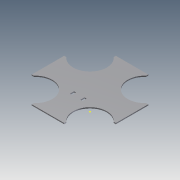
# Autodesk Inventor part: base bottom
Saved by Autodesk Inventor 2011 (Build 150239000, 239)
## iProperties
Created: 2011-07-30
Part Number: base bottom
Document SubType Name: Modeling
Designer: adowning
Density: 1 g/cm^3
Author: adowning
Autodesk Inventor part; units mm, degrees
ref_plane "YZ Plane" through (0, 0, 0) normal (1, 0, 0) x (0, 1, 0)
ref_plane "XZ Plane" through (0, 0, 0) normal (0, 1, 0) x (-1, 0, 0)
ref_plane "XY Plane" through (0, 0, 0) normal (0, 0, 1) x (1, 0, 0)
sketch "Sketch1" plane through (0, 0, 0) normal (0, 0, 1) x (1, 0, 0)
  point P0 (0, 0)
sketch "Sketch2" plane through (0, 0, 0) normal (0, 1, 0) x (-1, 0, 0)
  line L0 (-144.440152, 144.440152) -> (363.559848, 144.440152)
  line L1 (363.559848, 144.440152) -> (363.559848, -363.559848)
  line L2 (363.559848, -363.559848) -> (-144.440152, -363.559848)
  line L3 (-144.440152, -363.559848) -> (-144.440152, 144.440152)
  line L4 (363.559848, -363.559848) -> (274.659848, -363.559848)
  line L5 (274.659848, -363.559848) -> (274.659848, -274.659848)
  line L6 (274.659848, -274.659848) -> (363.559848, -274.659848)
  line L7 (363.559848, -274.659848) -> (363.559848, -363.559848)
  line L8 (-144.440152, -363.559848) -> (-55.540152, -363.559848)
  line L9 (-55.540152, -363.559848) -> (-55.540152, -274.659848)
  line L10 (-55.540152, -274.659848) -> (-144.440152, -274.659848)
  line L11 (-144.440152, -274.659848) -> (-144.440152, -363.559848)
  line L12 (-144.440152, 144.440152) -> (-55.540152, 144.440152)
  line L13 (-55.540152, 144.440152) -> (-55.540152, 55.540152)
  line L14 (-55.540152, 55.540152) -> (-144.440152, 55.540152)
  line L15 (-144.440152, 55.540152) -> (-144.440152, 144.440152)
  line L16 (363.559848, 144.440152) -> (274.659848, 144.440152)
  line L17 (274.659848, 144.440152) -> (274.659848, 55.540152)
  line L18 (274.659848, 55.540152) -> (363.559848, 55.540152)
  line L19 (363.559848, 55.540152) -> (363.559848, 144.440152)
  line L20 (363.559848, -363.559848) -> (173.059848, -363.559848)
  line L21 (173.059848, -363.559848) -> (173.059848, -173.059848)
  line L22 (173.059848, -173.059848) -> (363.559848, -173.059848)
  line L23 (363.559848, -173.059848) -> (363.559848, -363.559848)
  line L24 (-144.440152, -363.559848) -> (46.059848, -363.559848)
  line L25 (46.059848, -363.559848) -> (46.059848, -173.059848)
  line L26 (46.059848, -173.059848) -> (-144.440152, -173.059848)
  line L27 (-144.440152, -173.059848) -> (-144.440152, -363.559848)
  line L28 (-144.440152, 144.440152) -> (46.059848, 144.440152)
  line L29 (46.059848, 144.440152) -> (46.059848, -46.059848)
  line L30 (46.059848, -46.059848) -> (-144.440152, -46.059848)
  line L31 (-144.440152, -46.059848) -> (-144.440152, 144.440152)
  line L32 (363.559848, 144.440152) -> (173.059848, 144.440152)
  line L33 (173.059848, 144.440152) -> (173.059848, -46.059848)
  line L34 (173.059848, -46.059848) -> (363.559848, -46.059848)
  line L35 (363.559848, -46.059848) -> (363.559848, 144.440152)
  circle A0 centre (-55.540152, -274.659848) radius 101.6
  circle A1 centre (-55.540152, 55.540152) radius 101.6
  circle A2 centre (274.659848, 55.540152) radius 101.6
  circle A3 centre (274.659848, -274.659848) radius 101.6
  point P0 (0, 0)
  dimension "d0" = 508
  dimension "d1" = 508
  dimension "d2" = 88.9
  dimension "d3" = 88.9
  dimension "d4" = 88.9
  dimension "d5" = 88.9
  dimension "d6" = 88.9
  dimension "d7" = 88.9
  dimension "d8" = 88.9
  dimension "d9" = 88.9
  dimension "d10" = 190.5
  dimension "d11" = 190.5
  dimension "d12" = 190.5
  dimension "d13" = 190.5
  dimension "d14" = 190.5
  dimension "d15" = 190.5
  constraints: 72 end point, 18 parallel, 9 horizontal, 9 perpendicular, 4 centre point, 4 coincident, 4 tangent
  measures "d0" distance of L1.end L2.end
  measures "d1" distance of L0.end L1.end
  measures "d2" distance of L5.end L6.end
  measures "d3" distance of L4.end L5.end
  measures "d4" distance of L10.end L9.end
  measures "d5" distance of L9.end L8.end
  measures "d6" distance of L13.end L14.end
  measures "d7" distance of L12.end L13.end
  measures "d8" distance of L18.end L17.end
  measures "d9" distance of L17.end L16.end
  measures "d10" distance of L21.end L22.end
  measures "d11" distance of L20.end L21.end
  measures "d12" distance of L26.end L25.end
  measures "d13" distance of L25.end L24.end
  measures "d14" distance of L29.end L30.end
  measures "d15" distance of L28.end L29.end
extrude "Extrusion1" add sketch "Sketch2" along normal blind 12.7 contours L0 L33 L34 L1 L22 L21 L2 L25 L26 L3 L30 L29
fillet "Fillet1" radius 101.6 4 edges at (-173.0598, 6.35, -46.0598) (-46.0598, 6.35, -46.0598) (-46.0598, 6.35, -173.0598) (-173.0598, 6.35, -173.0598)
sketch "Sketch3" plane through (0, 12.7, 0) normal (0, 1, 0) x (1, 0, 0)
  line L0 (55.540152, 46.059848) -> (144.440152, 46.059848)
  line L1 (144.440152, 173.059848) -> (144.440152, 46.059848)
  line L2 (144.440152, 173.059848) -> (55.540152, 173.059848)
  arc A0 (-46.059848, 274.659848) -> (55.540152, 173.059848) centre (55.540152, 274.659848) ccw
  line L3 (-46.059848, 274.659848) -> (-46.059848, 363.559848)
  line L4 (-173.059848, 363.559848) -> (-46.059848, 363.559848)
  line L5 (-173.059848, 363.559848) -> (-173.059848, 274.659848)
  arc A1 (-274.659848, 173.059848) -> (-173.059848, 274.659848) centre (-274.659848, 274.659848) ccw
  line L6 (-274.659848, 173.059848) -> (-363.559848, 173.059848)
  line L7 (-363.559848, 46.059848) -> (-363.559848, 173.059848)
  line L8 (-363.559848, 46.059848) -> (-274.659848, 46.059848)
  arc A2 (-173.059848, -55.540152) -> (-274.659848, 46.059848) centre (-274.659848, -55.540152) ccw
  line L9 (-173.059848, -55.540152) -> (-173.059848, -144.440152)
  line L10 (-46.059848, -144.440152) -> (-173.059848, -144.440152)
  line L11 (-46.059848, -144.440152) -> (-46.059848, -55.540152)
  arc A3 (55.540152, 46.059848) -> (-46.059848, -55.540152) centre (55.540152, -55.540152) ccw
  circle A4 centre (55.540152, 274.659848) radius 101.6
  circle A5 centre (55.540152, -55.540152) radius 101.6
  circle A6 centre (-274.659848, -55.540152) radius 101.6
  circle A7 centre (-274.659848, 274.659848) radius 101.6
  line L12 (-46.059848, -144.440152) -> (6.353264, -144.440152)
  line L13 (-173.059848, -144.440152) -> (-225.472959, -144.440152)
  line L14 (-173.059848, 363.559848) -> (-225.472959, 363.559848)
  line L15 (-46.059848, 363.559848) -> (6.353264, 363.559848)
  line L16 (-173.059848, 363.559848) -> (-173.059848, 274.659848)
  line L17 (-46.059848, 363.559848) -> (-46.059848, 274.659848)
  line L18 (-46.059848, -144.440152) -> (-46.059848, -55.540152)
  line L19 (-173.059848, -144.440152) -> (-173.059848, -55.540152)
  line L20 (144.440152, 173.059848) -> (144.440152, 225.472959)
  line L21 (144.440152, 46.059848) -> (144.440152, -6.353264)
  line L22 (-363.559848, 46.059848) -> (-363.559848, -6.353264)
  line L23 (-363.559848, 173.059848) -> (-363.559848, 225.472959)
  line L24 (-363.559848, 173.059848) -> (-274.659848, 173.059848)
  line L25 (-363.559848, 46.059848) -> (-274.659848, 46.059848)
  line L26 (144.440152, 173.059848) -> (55.540152, 173.059848)
  line L27 (144.440152, 46.059848) -> (55.540152, 46.059848)
  point P0 (0, 0)
  constraints: 32 end point, 12 point on circle, 8 collinear, 8 tangent, 4 centre point, 4 coincident, 4 concentric, 4 point on line, 3 parallel, 1 perpendicular
extrude "Extrusion2" add sketch "Sketch3" against normal blind 12.7 contours A3 L11 L10 L9 A2 L8 L7 L6 A1 L5 L4 L3 A0 L2 L1 L0 | L0 L21 A5 | A5 L12 L11 | L13 A6 L9 | A6 L22 L8 | L5 A7 L14 | L23 A7 L6
sketch "Sketch4" plane through (0, 12.7, 0) normal (0, 1, 0) x (1, 0, 0)
  line L0 (144.440152, -6.353264) -> (144.440152, 173.059848)
  line L1 (144.440152, 173.059848) -> (55.540152, 173.059848)
  arc A0 (-46.059848, 274.659848) -> (55.540152, 173.059848) centre (55.540152, 274.659848) ccw
  line L2 (-46.059848, 274.659848) -> (-46.059848, 363.559848)
  line L3 (-225.472959, 363.559848) -> (-46.059848, 363.559848)
  arc A1 (-363.559848, 225.472959) -> (-225.472959, 363.559848) centre (-274.659848, 274.659848) ccw
  line L4 (-363.559848, -6.353264) -> (-363.559848, 225.472959)
  arc A2 (-225.472959, -144.440152) -> (-363.559848, -6.353264) centre (-274.659848, -55.540152) ccw
  line L5 (6.353264, -144.440152) -> (-225.472959, -144.440152)
  arc A3 (144.440152, -6.353264) -> (6.353264, -144.440152) centre (55.540152, -55.540152) ccw
  circle A4 centre (55.540152, 274.659848) radius 101.6
  line L6 (-46.059848, 363.559848) -> (6.353264, 363.559848)
  line L7 (144.440152, 173.059848) -> (144.440152, 225.472959)
  line L8 (144.440152, 173.059848) -> (55.540152, 173.059848)
  line L9 (-46.059848, 363.559848) -> (-46.059848, 274.659848)
  point P0 (0, 0)
  constraints: 8 end point, 4 point on circle, 2 point on line, 1 centre point, 1 coincident, 1 concentric, 1 parallel, 1 perpendicular
extrude "Extrusion3" add sketch "Sketch4" against normal blind 12.7 contours A3 L5 A2 L4 A1 L3 L2 A0 L1 L0 | L1 A4 L7 | L2 L6 A4
sketch "Sketch5" plane through (0, 12.7, 0) normal (0, 1, 0) x (1, 0, 0)
  line L0 (144.440152, -6.353264) -> (144.440152, 225.472959)
  line L1 (-363.559848, -6.353264) -> (-363.559848, 225.472959)
  line L2 (6.353264, -144.440152) -> (-225.472959, -144.440152)
  line L3 (-363.559848, 225.472959) -> (-363.559848, 109.560059)
  line L4 (-225.472959, -144.440152) -> (-109.560059, -144.440152)
  line L5 (144.440152, -6.353264) -> (144.440152, 109.559848)
  line L6 (144.440152, 109.559848) -> (144.440152, 43.519848)
  line L7 (-363.559848, 109.560059) -> (-363.559848, 43.519848)
  line L8 (-109.560059, -144.440152) -> (-175.600059, -144.440152)
  line L9 (-175.600059, -144.440152) -> (-43.520059, -144.440152)
  line L10 (-363.559848, 43.519848) -> (-363.559848, 175.599848)
  line L11 (-175.600059, -144.440152) -> (-181.950059, -144.440152)
  line L12 (-181.950059, -144.440152) -> (-181.950059, -138.090152)
  line L13 (-181.950059, -138.090152) -> (-175.600059, -138.090152)
  line L14 (-175.600059, -138.090152) -> (-175.600059, -144.440152)
  line L15 (-43.520059, -144.440152) -> (-37.170059, -144.440152)
  line L16 (-37.170059, -144.440152) -> (-37.170059, -138.090152)
  line L17 (-37.170059, -138.090152) -> (-43.520059, -138.090152)
  line L18 (-43.520059, -138.090152) -> (-43.520059, -144.440152)
  line L19 (144.440152, 43.519848) -> (138.090152, 43.519848)
  line L20 (138.090152, 43.519848) -> (138.090152, 37.169848)
  line L21 (138.090152, 37.169848) -> (144.440152, 37.169848)
  line L22 (144.440152, 37.169848) -> (144.440152, 43.519848)
  line L23 (144.440152, 43.519848) -> (144.440152, 175.599848)
  line L24 (-363.559848, 43.519848) -> (-357.209848, 43.519848)
  line L25 (-357.209848, 43.519848) -> (-357.209848, 37.169848)
  line L26 (-357.209848, 37.169848) -> (-363.559848, 37.169848)
  line L27 (-363.559848, 37.169848) -> (-363.559848, 43.519848)
  line L28 (-363.559848, 175.599848) -> (-357.209848, 175.599848)
  line L29 (-357.209848, 175.599848) -> (-357.209848, 181.949848)
  line L30 (-357.209848, 181.949848) -> (-363.559848, 181.949848)
  line L31 (-363.559848, 181.949848) -> (-363.559848, 175.599848)
  line L32 (144.440152, 175.599848) -> (138.090152, 175.599848)
  line L33 (138.090152, 175.599848) -> (138.090152, 181.949848)
  line L34 (138.090152, 181.949848) -> (144.440152, 181.949848)
  line L35 (144.440152, 181.949848) -> (144.440152, 175.599848)
  point P0 (0, 0)
  dimension "d23" = 115.9129
  dimension "d24" = 115.9129
  dimension "d25" = 66.04
  dimension "d26" = 66.04
  dimension "d27" = 132.08
  dimension "d28" = 132.08
  dimension "d29" = 6.35
  dimension "d30" = 6.35
  dimension "d31" = 6.35
  dimension "d32" = 6.35
  dimension "d33" = 6.35
  dimension "d34" = 6.35
  dimension "d35" = 132.08
  dimension "d36" = 6.35
  dimension "d37" = 6.35
  dimension "d38" = 6.35
  dimension "d39" = 6.35
  dimension "d40" = 6.35
  dimension "d41" = 6.35
  constraints: 66 end point, 12 parallel, 8 point on line, 6 horizontal, 6 perpendicular, 1 midpoint
  measures "d23" distance of L1.end L3.end
  measures "d24" distance of L2.end L4.end
  measures "d25" distance of L5.end L6.end
  measures "d26" distance of L4.end L8.end
  measures "d27" distance of L8.end L9.end
  measures "d28" distance of L7.end L10.end
  measures "d29" distance of L12.end L13.end
  measures "d30" distance of L11.end L12.end
  measures "d31" distance of L17.end L16.end
  measures "d32" distance of L16.end L15.end
  measures "d33" distance of L21.end L20.end
  measures "d34" distance of L20.end L19.end
  measures "d35" distance of L6.end L23.end
  measures "d36" distance of L25.end L26.end
  measures "d37" distance of L24.end L25.end
  measures "d38" distance of L30.end L29.end
  measures "d39" distance of L29.end L28.end
  measures "d40" distance of L33.end L34.end
  measures "d41" distance of L32.end L33.end
extrude "Extrusion4" cut sketch "Sketch5" against normal blind 25.4
sketch "Sketch6" plane through (0, 12.7, 0) normal (0, 1, 0) x (1, 0, 0)
  line L0 (-175.600059, -138.090152) -> (-175.600059, -144.440152)
  line L1 (-43.520059, -144.440152) -> (-175.600059, -144.440152)
  line L2 (-43.520059, -144.440152) -> (-43.520059, -138.090152)
  line L3 (-43.520059, -138.090152) -> (-37.170059, -138.090152)
  line L4 (-37.170059, -138.090152) -> (-37.170059, -144.440152)
  line L5 (6.353264, -144.440152) -> (-37.170059, -144.440152)
  arc A0 (144.440152, -6.353264) -> (6.353264, -144.440152) centre (55.540152, -55.540152) ccw
  line L6 (144.440152, -6.353264) -> (144.440152, 37.169848)
  line L7 (144.440152, 37.169848) -> (138.090152, 37.169848)
  line L8 (138.090152, 37.169848) -> (138.090152, 43.519848)
  line L9 (138.090152, 43.519848) -> (144.440152, 43.519848)
  line L10 (144.440152, 43.519848) -> (144.440152, 175.599848)
  line L11 (144.440152, 175.599848) -> (138.090152, 175.599848)
  line L12 (138.090152, 175.599848) -> (138.090152, 181.949848)
  line L13 (138.090152, 181.949848) -> (144.440152, 181.949848)
  line L14 (144.440152, 181.949848) -> (144.440152, 225.472959)
  arc A1 (6.353264, 363.559848) -> (144.440152, 225.472959) centre (55.540152, 274.659848) ccw
  line L15 (-225.472959, 363.559848) -> (6.353264, 363.559848)
  arc A2 (-363.559848, 225.472959) -> (-225.472959, 363.559848) centre (-274.659848, 274.659848) ccw
  line L16 (-363.559848, 181.949848) -> (-363.559848, 225.472959)
  line L17 (-363.559848, 181.949848) -> (-357.209848, 181.949848)
  line L18 (-357.209848, 181.949848) -> (-357.209848, 175.599848)
  line L19 (-357.209848, 175.599848) -> (-363.559848, 175.599848)
  line L20 (-363.559848, 43.519848) -> (-363.559848, 175.599848)
  line L21 (-363.559848, 43.519848) -> (-357.209848, 43.519848)
  line L22 (-357.209848, 43.519848) -> (-357.209848, 37.169848)
  line L23 (-357.209848, 37.169848) -> (-363.559848, 37.169848)
  line L24 (-363.559848, -6.353264) -> (-363.559848, 37.169848)
  arc A3 (-225.472959, -144.440152) -> (-363.559848, -6.353264) centre (-274.659848, -55.540152) ccw
  line L25 (-181.950059, -144.440152) -> (-225.472959, -144.440152)
  line L26 (-181.950059, -144.440152) -> (-181.950059, -138.090152)
  line L27 (-181.950059, -138.090152) -> (-175.600059, -138.090152)
  point P0 (0, 0)
extrude "Extrusion5" cut sketch "Sketch6" against normal blind 6.35
sketch "Sketch7" plane through (0, 6.35, 0) normal (0, 1, 0) x (1, 0, 0)
  line L0 (-43.520059, -144.440152) -> (-175.600059, -144.440152)
  line L1 (144.440152, 175.599848) -> (144.440152, 43.519848)
  line L2 (-363.559848, 43.519848) -> (-363.559848, 175.599848)
  line L3 (-363.559848, 175.599848) -> (-363.559848, 137.499848)
  line L4 (-363.559848, 43.519848) -> (-363.559848, 81.619848)
  line L5 (-175.600059, -144.440152) -> (-137.500059, -144.440152)
  line L6 (-43.520059, -144.440152) -> (-81.620059, -144.440152)
  line L7 (144.440152, 43.519848) -> (144.440152, 81.619848)
  line L8 (144.440152, 175.599848) -> (144.440152, 137.499848)
  line L9 (-363.559848, 81.619848) -> (-357.209848, 81.619848)
  line L10 (-357.209848, 81.619848) -> (-357.209848, 87.969848)
  line L11 (-357.209848, 87.969848) -> (-363.559848, 87.969848)
  line L12 (-363.559848, 87.969848) -> (-363.559848, 81.619848)
  line L13 (-363.559848, 137.499848) -> (-357.209848, 137.499848)
  line L14 (-357.209848, 137.499848) -> (-357.209848, 131.149848)
  line L15 (-357.209848, 131.149848) -> (-363.559848, 131.149848)
  line L16 (-363.559848, 131.149848) -> (-363.559848, 137.499848)
  line L17 (-137.500059, -144.440152) -> (-131.150059, -144.440152)
  line L18 (-131.150059, -144.440152) -> (-131.150059, -138.090152)
  line L19 (-131.150059, -138.090152) -> (-137.500059, -138.090152)
  line L20 (-137.500059, -138.090152) -> (-137.500059, -144.440152)
  line L21 (-81.620059, -144.440152) -> (-87.970059, -144.440152)
  line L22 (-87.970059, -144.440152) -> (-87.970059, -138.090152)
  line L23 (-87.970059, -138.090152) -> (-81.620059, -138.090152)
  line L24 (-81.620059, -138.090152) -> (-81.620059, -144.440152)
  line L25 (144.440152, 81.619848) -> (138.090152, 81.619848)
  line L26 (138.090152, 81.619848) -> (138.090152, 87.969848)
  line L27 (138.090152, 87.969848) -> (144.440152, 87.969848)
  line L28 (144.440152, 87.969848) -> (144.440152, 81.619848)
  line L29 (144.440152, 137.499848) -> (138.090152, 137.499848)
  line L30 (138.090152, 137.499848) -> (138.090152, 131.149848)
  line L31 (138.090152, 131.149848) -> (144.440152, 131.149848)
  line L32 (144.440152, 131.149848) -> (144.440152, 137.499848)
  point P0 (0, 0)
  dimension "d46" = 38.1
  dimension "d47" = 38.1
  dimension "d48" = 38.1
  dimension "d49" = 38.1
  dimension "d50" = 6.35
  dimension "d51" = 6.35
  dimension "d52" = 6.35
  dimension "d53" = 6.35
  dimension "d54" = 6.35
  dimension "d55" = 6.35
  dimension "d56" = 6.35
  dimension "d57" = 6.35
  dimension "d58" = 6.35
  dimension "d59" = 6.35
  dimension "d60" = 6.35
  dimension "d61" = 6.35
  constraints: 60 end point, 12 parallel, 6 horizontal, 6 perpendicular, 6 point on line
  measures "d46" distance of L2.end L3.end
  measures "d47" distance of L2.start L4.end
  measures "d48" distance of L0.end L5.end
  measures "d49" distance of L0.start L6.end
  measures "d50" distance of L11.end L10.end
  measures "d51" distance of L10.end L9.end
  measures "d52" distance of L14.end L15.end
  measures "d53" distance of L13.end L14.end
  measures "d54" distance of L19.end L18.end
  measures "d55" distance of L18.end L17.end
  measures "d56" distance of L22.end L23.end
  measures "d57" distance of L21.end L22.end
  measures "d58" distance of L26.end L27.end
  measures "d59" distance of L25.end L26.end
  measures "d60" distance of L31.end L30.end
  measures "d61" distance of L30.end L29.end
extrude "Extrusion6" cut sketch "Sketch7" against normal blind 6.35
sketch "Sketch8" plane through (0, 6.35, 0) normal (0, 1, 0) x (1, 0, 0)
  line L0 (-225.472959, 363.559848) -> (6.353264, 363.559848)
  line L1 (-225.472959, 363.559848) -> (-187.372959, 363.559848)
  line L2 (6.353264, 363.559848) -> (-31.746736, 363.559848)
  line L3 (-31.746736, 363.559848) -> (-31.746736, 357.209848)
  line L4 (6.353264, 363.559848) -> (-6.346736, 363.559848)
  line L5 (-31.746736, 357.209848) -> (-57.146736, 357.209848)
  line L6 (-57.146736, 357.209848) -> (-57.146736, 363.559848)
  line L7 (-187.372959, 363.559848) -> (-187.372959, 357.209848)
  line L8 (-187.372959, 357.209848) -> (-161.972959, 357.209848)
  line L9 (-161.972959, 357.209848) -> (-161.972959, 363.559848)
  line L10 (-161.972959, 363.559848) -> (-136.572959, 363.559848)
  line L11 (-136.572959, 363.559848) -> (-136.572959, 357.209848)
  line L12 (-57.146736, 363.559848) -> (-82.546736, 363.559848)
  line L13 (-82.546736, 363.559848) -> (-82.546736, 357.209848)
  line L14 (-82.546736, 357.209848) -> (-95.246736, 357.209848)
  line L15 (-95.246736, 357.209848) -> (-95.246736, 363.559848)
  line L16 (-136.572959, 357.209848) -> (-123.872959, 357.209848)
  line L17 (-123.872959, 357.209848) -> (-123.872959, 363.559848)
  point P0 (0, 0)
  dimension "d64" = 38.1
  dimension "d65" = 38.1
  dimension "d66" = 6.35
  dimension "d67" = 12.7
  dimension "d68" = 25.4
  dimension "d69" = 6.35
  dimension "d70" = 25.4
  dimension "d71" = 25.4
  dimension "d72" = 25.4
  dimension "d73" = 12.7
  dimension "d74" = 12.7
  constraints: 34 end point, 7 vertical, 3 perpendicular, 2 parallel, 1 point on line, 9 other
  measures "d64" distance of L1.start L1.end
  measures "d65" distance of L2.start L2.end
  measures "d66" distance of L2.end L3.end
  measures "d67" distance of L2.start L4.end
  measures "d68" distance of L3.end L5.end
  measures "d69" distance of L1.end L7.end
  measures "d70" distance of L7.end L8.end
  measures "d71" distance of L9.end L10.end
  measures "d72" distance of L6.end L12.end
  measures "d73" distance of L13.end L14.end
  measures "d74" distance of L11.end L16.end
extrude "Extrusion7" cut sketch "Sketch8" against normal blind 25.4
sketch "Sketch9" plane through (0, 6.35, 0) normal (0, 1, 0) x (1, 0, 0)
  line L0 (-31.746736, 363.559848) -> (-31.746736, 357.209848)
  line L1 (-31.746736, 357.209848) -> (-57.146736, 357.209848)
  line L2 (-57.146736, 357.209848) -> (-57.146736, 363.559848)
  line L3 (-82.546736, 363.559848) -> (-57.146736, 363.559848)
  line L4 (-82.546736, 363.559848) -> (-82.546736, 357.209848)
  line L5 (-82.546736, 357.209848) -> (-95.246736, 357.209848)
  line L6 (-95.246736, 357.209848) -> (-95.246736, 363.559848)
  line L7 (-123.872959, 363.559848) -> (-95.246736, 363.559848)
  line L8 (-123.872959, 363.559848) -> (-123.872959, 357.209848)
  line L9 (-123.872959, 357.209848) -> (-136.572959, 357.209848)
  line L10 (-136.572959, 357.209848) -> (-136.572959, 363.559848)
  line L11 (-161.972959, 363.559848) -> (-136.572959, 363.559848)
  line L12 (-161.972959, 363.559848) -> (-161.972959, 357.209848)
  line L13 (-161.972959, 357.209848) -> (-187.372959, 357.209848)
  line L14 (-187.372959, 357.209848) -> (-187.372959, 363.559848)
  line L15 (-225.472959, 363.559848) -> (-187.372959, 363.559848)
  arc A0 (-363.559848, 225.472959) -> (-225.472959, 363.559848) centre (-274.659848, 274.659848) ccw
  line L16 (-363.559848, 181.949848) -> (-363.559848, 225.472959)
  line L17 (-357.209848, 181.949848) -> (-363.559848, 181.949848)
  line L18 (-357.209848, 175.599848) -> (-357.209848, 181.949848)
  line L19 (-363.559848, 175.599848) -> (-357.209848, 175.599848)
  line L20 (-363.559848, 137.499848) -> (-363.559848, 175.599848)
  line L21 (-363.559848, 137.499848) -> (-357.209848, 137.499848)
  line L22 (-357.209848, 137.499848) -> (-357.209848, 131.149848)
  line L23 (-357.209848, 131.149848) -> (-363.559848, 131.149848)
  line L24 (-363.559848, 87.969848) -> (-363.559848, 131.149848)
  line L25 (-363.559848, 87.969848) -> (-357.209848, 87.969848)
  line L26 (-357.209848, 87.969848) -> (-357.209848, 81.619848)
  line L27 (-357.209848, 81.619848) -> (-363.559848, 81.619848)
  line L28 (-363.559848, 43.519848) -> (-363.559848, 81.619848)
  line L29 (-357.209848, 43.519848) -> (-363.559848, 43.519848)
  line L30 (-357.209848, 37.169848) -> (-357.209848, 43.519848)
  line L31 (-363.559848, 37.169848) -> (-357.209848, 37.169848)
  line L32 (-363.559848, -6.353264) -> (-363.559848, 37.169848)
  arc A1 (-225.472959, -144.440152) -> (-363.559848, -6.353264) centre (-274.659848, -55.540152) ccw
  line L33 (-181.950059, -144.440152) -> (-225.472959, -144.440152)
  line L34 (-181.950059, -138.090152) -> (-181.950059, -144.440152)
  line L35 (-175.600059, -138.090152) -> (-181.950059, -138.090152)
  line L36 (-175.600059, -144.440152) -> (-175.600059, -138.090152)
  line L37 (-137.500059, -144.440152) -> (-175.600059, -144.440152)
  line L38 (-137.500059, -144.440152) -> (-137.500059, -138.090152)
  line L39 (-137.500059, -138.090152) -> (-131.150059, -138.090152)
  line L40 (-131.150059, -138.090152) -> (-131.150059, -144.440152)
  line L41 (-87.970059, -144.440152) -> (-131.150059, -144.440152)
  line L42 (-87.970059, -144.440152) -> (-87.970059, -138.090152)
  line L43 (-87.970059, -138.090152) -> (-81.620059, -138.090152)
  line L44 (-81.620059, -138.090152) -> (-81.620059, -144.440152)
  line L45 (-43.520059, -144.440152) -> (-81.620059, -144.440152)
  line L46 (-43.520059, -138.090152) -> (-43.520059, -144.440152)
  line L47 (-37.170059, -138.090152) -> (-43.520059, -138.090152)
  line L48 (-37.170059, -144.440152) -> (-37.170059, -138.090152)
  line L49 (6.353264, -144.440152) -> (-37.170059, -144.440152)
  arc A2 (144.440152, -6.353264) -> (6.353264, -144.440152) centre (55.540152, -55.540152) ccw
  line L50 (144.440152, 37.169848) -> (144.440152, -6.353264)
  line L51 (138.090152, 37.169848) -> (144.440152, 37.169848)
  line L52 (138.090152, 43.519848) -> (138.090152, 37.169848)
  line L53 (144.440152, 43.519848) -> (138.090152, 43.519848)
  line L54 (144.440152, 81.619848) -> (144.440152, 43.519848)
  line L55 (144.440152, 81.619848) -> (138.090152, 81.619848)
  line L56 (138.090152, 81.619848) -> (138.090152, 87.969848)
  line L57 (138.090152, 87.969848) -> (144.440152, 87.969848)
  line L58 (144.440152, 131.149848) -> (144.440152, 87.969848)
  line L59 (144.440152, 131.149848) -> (138.090152, 131.149848)
  line L60 (138.090152, 131.149848) -> (138.090152, 137.499848)
  line L61 (138.090152, 137.499848) -> (144.440152, 137.499848)
  line L62 (144.440152, 175.599848) -> (144.440152, 137.499848)
  line L63 (138.090152, 175.599848) -> (144.440152, 175.599848)
  line L64 (138.090152, 181.949848) -> (138.090152, 175.599848)
  line L65 (144.440152, 181.949848) -> (138.090152, 181.949848)
  line L66 (144.440152, 225.472959) -> (144.440152, 181.949848)
  arc A3 (6.353264, 363.559848) -> (144.440152, 225.472959) centre (55.540152, 274.659848) ccw
  line L67 (-31.746736, 363.559848) -> (6.353264, 363.559848)
  line L68 (-187.372959, 363.559848) -> (-31.746736, 363.559848)
  point P0 (0, 0)
  constraints: 2 end point, 1 collinear
extrude "Extrusion8" add sketch "Sketch9" against normal blind 6.35 contours L0 L1 L2 L68 | L4 L5 L6 L68 | L8 L9 L10 L68 | L12 L13 L14 L68
sketch "Sketch10" plane through (0, 6.35, 0) normal (0, 1, 0) x (1, 0, 0)
  line L0 (-225.472959, 363.559848) -> (6.353264, 363.559848)
  line L1 (-225.472959, 363.559848) -> (-109.560059, 363.559848)
  line L2 (-109.560059, 363.559848) -> (-94.320059, 363.559848)
  line L3 (-94.320059, 363.559848) -> (-124.800059, 363.559848)
  line L4 (-124.800059, 363.559848) -> (-137.500059, 363.559848)
  line L5 (-137.500059, 363.559848) -> (-137.500059, 357.209848)
  line L6 (-137.500059, 357.209848) -> (-124.800059, 357.209848)
  line L7 (-124.800059, 357.209848) -> (-124.800059, 363.559848)
  line L8 (-94.320059, 363.559848) -> (-81.620059, 363.559848)
  line L9 (-81.620059, 363.559848) -> (-81.620059, 357.209848)
  line L10 (-81.620059, 357.209848) -> (-94.320059, 357.209848)
  line L11 (-94.320059, 357.209848) -> (-94.320059, 363.559848)
  line L12 (-81.620059, 357.209848) -> (-56.220059, 357.209848)
  line L13 (-56.220059, 357.209848) -> (-30.820059, 357.209848)
  line L14 (-30.820059, 357.209848) -> (-30.820059, 363.559848)
  line L15 (-30.820059, 363.559848) -> (-56.220059, 363.559848)
  line L16 (-56.220059, 363.559848) -> (-56.220059, 357.209848)
  line L17 (-141.759572, 357.209848) -> (-167.159572, 357.209848)
  line L18 (-167.159572, 357.209848) -> (-192.559572, 357.209848)
  line L19 (-192.559572, 357.209848) -> (-192.559572, 363.559848)
  line L20 (-192.559572, 363.559848) -> (-167.159572, 363.559848)
  line L21 (-167.159572, 363.559848) -> (-167.159572, 357.209848)
  point P0 (0, 0)
  dimension "d79" = 115.9129
  dimension "d80" = 15.24
  dimension "d81" = 30.48
  dimension "d82" = 12.7
  dimension "d83" = 6.35
  dimension "d84" = 12.7
  dimension "d85" = 6.35
  dimension "d86" = 25.4
  dimension "d87" = 25.4
  dimension "d88" = 25.4
  dimension "d89" = 25.4
  constraints: 42 end point, 8 parallel, 6 perpendicular, 5 point on line, 4 horizontal
  measures "d79" distance of L0.start L1.end
  measures "d80" distance of L1.end L2.end
  measures "d81" distance of L2.end L3.end
  measures "d82" distance of L6.end L5.end
  measures "d83" distance of L5.end L4.end
  measures "d84" distance of L9.end L10.end
  measures "d85" distance of L8.end L9.end
  measures "d86" distance of L9.end L12.end
  measures "d87" distance of L15.end L14.end
  measures "d88" distance of L17.start L17.end
  measures "d89" distance of L19.end L20.end
extrude "Extrusion9" cut sketch "Sketch10" against normal blind 6.35 contours L0 L21 L18 L19 | L0 L7 L6 L5 | L0 L9 L10 L11 | L0 L14 L13 L16
sketch "Sketch11" plane through (0, 6.35, 0) normal (0, 1, 0) x (1, 0, 0)
  line L0 (-167.159572, 363.559848) -> (-167.159572, 357.209848)
  line L1 (-167.159572, 357.209848) -> (-192.559572, 357.209848)
  line L2 (-192.559572, 357.209848) -> (-192.559572, 363.559848)
  line L3 (-167.159572, 363.559848) -> (-137.500059, 363.559848)
  line L4 (-167.159572, 363.559848) -> (-192.559572, 363.559848)
  point P0 (0, 0)
  constraints: 2 end point, 1 collinear
extrude "Extrusion10" add sketch "Sketch11" against normal blind 6.35
sketch "Sketch12" plane through (0, 6.35, 0) normal (0, 1, 0) x (1, 0, 0)
  line L0 (-225.472959, 363.559848) -> (-137.500059, 363.559848)
  line L1 (-137.500059, 363.559848) -> (-162.900059, 363.559848)
  line L2 (-162.900059, 363.559848) -> (-188.300059, 363.559848)
  line L3 (-188.300059, 363.559848) -> (-188.300059, 357.209848)
  line L4 (-188.300059, 357.209848) -> (-162.900059, 357.209848)
  line L5 (-162.900059, 357.209848) -> (-162.900059, 363.559848)
  point P0 (0, 0)
  dimension "d94" = 25.4
  dimension "d95" = 25.4
  constraints: 10 end point, 2 parallel, 1 horizontal, 1 perpendicular, 1 point on line
  measures "d94" distance of L0.end L1.end
  measures "d95" distance of L4.end L3.end
extrude "Extrusion11" cut sketch "Sketch12" against normal blind 6.35
fillet "Fillet2" radius 3.175 1 edges at (6.3533, 3.175, -363.5598)
fillet "Fillet3" radius 3.175 1 edges at (-225.473, 3.175, -363.5598)
fillet "Fillet4" radius 3.175 6 edges at (144.4402, 3.175, 6.3533) (144.4402, 3.175, -225.473) (6.3533, 3.175, 144.4402) (-225.473, 3.175, 144.4402) (-363.5598, 3.175, 6.3533) (-363.5598, 3.175, -225.473)
sketch "Sketch13" plane through (0, 0, 0) normal (0, -1, 0) x (1, 0, 0)
  line L0 (-363.559848, -37.169848) -> (-363.559848, -4.701237)
  line L1 (-363.559848, -81.619848) -> (-363.559848, -43.519848)
  line L2 (-357.209848, -87.969848) -> (-363.559848, -87.969848)
  line L3 (-363.559848, -131.149848) -> (-363.559848, -87.969848)
  line L4 (-357.209848, -181.949848) -> (-363.559848, -181.949848)
  line L5 (-363.559848, -214.418458) -> (-363.559848, -181.949848)
  line L6 (-357.209848, -181.949848) -> (-363.559848, -181.949848)
  line L7 (-363.559848, -181.949848) -> (-363.559848, -188.299848)
  line L8 (-363.559848, -188.299848) -> (-357.209848, -188.299848)
  line L9 (-357.209848, -188.299848) -> (-357.209848, -181.949848)
  line L10 (-357.209848, -137.499848) -> (-363.559848, -137.499848)
  line L11 (-363.559848, -137.499848) -> (-363.559848, -143.849848)
  line L12 (-363.559848, -143.849848) -> (-357.209848, -143.849848)
  line L13 (-357.209848, -143.849848) -> (-357.209848, -137.499848)
  line L14 (-357.209848, -131.149848) -> (-363.559848, -131.149848)
  line L15 (-363.559848, -131.149848) -> (-363.559848, -124.799848)
  line L16 (-363.559848, -124.799848) -> (-357.209848, -124.799848)
  line L17 (-357.209848, -124.799848) -> (-357.209848, -131.149848)
  line L18 (-357.209848, -87.969848) -> (-363.559848, -87.969848)
  line L19 (-363.559848, -87.969848) -> (-363.559848, -94.319848)
  line L20 (-363.559848, -94.319848) -> (-357.209848, -94.319848)
  line L21 (-357.209848, -94.319848) -> (-357.209848, -87.969848)
  line L22 (-357.209848, -81.619848) -> (-363.559848, -81.619848)
  line L23 (-363.559848, -81.619848) -> (-363.559848, -75.269848)
  line L24 (-363.559848, -75.269848) -> (-357.209848, -75.269848)
  line L25 (-357.209848, -75.269848) -> (-357.209848, -81.619848)
  line L26 (-357.209848, -37.169848) -> (-363.559848, -37.169848)
  line L27 (-363.559848, -37.169848) -> (-363.559848, -30.819848)
  line L28 (-363.559848, -30.819848) -> (-357.209848, -30.819848)
  line L29 (-357.209848, -30.819848) -> (-357.209848, -37.169848)
  point P0 (0, 0)
  dimension "d101" = 6.35
  dimension "d102" = 6.35
  dimension "d103" = 6.35
  dimension "d104" = 6.35
  dimension "d105" = 6.35
  dimension "d106" = 6.35
  dimension "d107" = 6.35
  constraints: 48 end point, 12 parallel, 6 horizontal, 6 perpendicular, 5 point on line
  measures "d101" distance of L7.end L6.end
  measures "d102" distance of L12.end L11.end
  measures "d103" distance of L11.end L10.end
  measures "d104" distance of L14.end L15.end
  measures "d105" distance of L19.end L18.end
  measures "d106" distance of L22.end L23.end
  measures "d107" distance of L26.end L27.end
extrude "Extrusion12" cut sketch "Sketch13" against normal blind 6.35
sketch "Sketch14" plane through (0, 6.35, 0) normal (0, 1, 0) x (1, 0, 0)
  line L0 (144.440152, 37.169848) -> (144.440152, 4.701237)
  line L1 (144.440152, 81.619848) -> (144.440152, 43.519848)
  line L2 (144.440152, 131.149848) -> (144.440152, 87.969848)
  line L3 (144.440152, 181.949848) -> (138.090152, 181.949848)
  line L4 (138.090152, 181.949848) -> (138.090152, 188.299848)
  line L5 (138.090152, 188.299848) -> (144.440152, 188.299848)
  line L6 (144.440152, 188.299848) -> (144.440152, 181.949848)
  line L7 (138.090152, 143.849848) -> (144.440152, 143.849848)
  line L8 (144.440152, 143.849848) -> (144.440152, 124.799848)
  line L9 (144.440152, 124.799848) -> (138.090152, 124.799848)
  line L10 (138.090152, 124.799848) -> (138.090152, 143.849848)
  line L11 (138.090152, 94.319848) -> (144.440152, 94.319848)
  line L12 (144.440152, 94.319848) -> (144.440152, 75.269848)
  line L13 (144.440152, 75.269848) -> (138.090152, 75.269848)
  line L14 (138.090152, 75.269848) -> (138.090152, 94.319848)
  line L15 (138.090152, 37.169848) -> (144.440152, 37.169848)
  line L16 (144.440152, 37.169848) -> (144.440152, 30.819848)
  line L17 (144.440152, 30.819848) -> (138.090152, 30.819848)
  line L18 (138.090152, 30.819848) -> (138.090152, 37.169848)
  line L19 (-181.950059, -144.440152) -> (-188.300059, -144.440152)
  line L20 (-188.300059, -144.440152) -> (-188.300059, -138.090152)
  line L21 (-188.300059, -138.090152) -> (-181.950059, -138.090152)
  line L22 (-181.950059, -138.090152) -> (-181.950059, -144.440152)
  line L23 (-131.150059, -144.440152) -> (-124.800059, -144.440152)
  line L24 (-124.800059, -144.440152) -> (-124.800059, -138.090152)
  line L25 (-124.800059, -138.090152) -> (-131.150059, -138.090152)
  line L26 (-131.150059, -138.090152) -> (-131.150059, -144.440152)
  line L27 (-137.500059, -144.440152) -> (-143.850059, -144.440152)
  line L28 (-143.850059, -144.440152) -> (-143.850059, -138.090152)
  line L29 (-143.850059, -138.090152) -> (-137.500059, -138.090152)
  line L30 (-137.500059, -138.090152) -> (-137.500059, -144.440152)
  line L31 (-87.970059, -144.440152) -> (-94.320059, -144.440152)
  line L32 (-94.320059, -144.440152) -> (-94.320059, -138.090152)
  line L33 (-94.320059, -138.090152) -> (-87.970059, -138.090152)
  line L34 (-87.970059, -138.090152) -> (-87.970059, -144.440152)
  line L35 (-81.620059, -144.440152) -> (-75.270059, -144.440152)
  line L36 (-75.270059, -144.440152) -> (-75.270059, -138.090152)
  line L37 (-75.270059, -138.090152) -> (-81.620059, -138.090152)
  line L38 (-81.620059, -138.090152) -> (-81.620059, -144.440152)
  line L39 (-37.170059, -144.440152) -> (-30.820059, -144.440152)
  line L40 (-30.820059, -144.440152) -> (-30.820059, -138.090152)
  line L41 (-30.820059, -138.090152) -> (-37.170059, -138.090152)
  line L42 (-37.170059, -138.090152) -> (-37.170059, -144.440152)
  point P0 (0, 0)
  dimension "d110" = 6.35
  dimension "d111" = 6.35
  constraints: 80 end point, 20 parallel, 10 horizontal, 10 perpendicular, 3 point on line
  measures "d110" distance of L28.end L29.end
  measures "d111" distance of L37.end L36.end
extrude "Extrusion13" cut sketch "Sketch14" against normal blind 6.35
sketch "Sketch15" plane through (0, 6.35, 0) normal (0, 1, 0) x (1, 0, 0)
  line L0 (138.090152, 188.299848) -> (144.440152, 188.299848)
  line L1 (144.440152, 214.418458) -> (144.440152, 188.299848)
  arc A0 (144.440152, 214.418458) -> (138.667425, 216.243955) centre (141.265152, 214.418458) ccw
  arc A1 (-2.87574, 357.78712) -> (138.667425, 216.243955) centre (55.540152, 274.659848) ccw
  arc A2 (-2.87574, 357.78712) -> (-4.701237, 363.559848) centre (-4.701237, 360.384848) ccw
  line L2 (-30.820059, 363.559848) -> (-4.701237, 363.559848)
  line L3 (-30.820059, 363.559848) -> (-30.820059, 357.209848)
  line L4 (-30.820059, 357.209848) -> (-56.220059, 357.209848)
  line L5 (-56.220059, 357.209848) -> (-56.220059, 363.559848)
  line L6 (-81.620059, 363.559848) -> (-56.220059, 363.559848)
  line L7 (-81.620059, 363.559848) -> (-81.620059, 357.209848)
  line L8 (-81.620059, 357.209848) -> (-94.320059, 357.209848)
  line L9 (-94.320059, 357.209848) -> (-94.320059, 363.559848)
  line L10 (-124.800059, 363.559848) -> (-94.320059, 363.559848)
  line L11 (-124.800059, 363.559848) -> (-124.800059, 357.209848)
  line L12 (-124.800059, 357.209848) -> (-137.500059, 357.209848)
  line L13 (-137.500059, 357.209848) -> (-137.500059, 363.559848)
  line L14 (-162.900059, 363.559848) -> (-137.500059, 363.559848)
  line L15 (-162.900059, 363.559848) -> (-162.900059, 357.209848)
  line L16 (-162.900059, 357.209848) -> (-188.300059, 357.209848)
  line L17 (-188.300059, 357.209848) -> (-188.300059, 363.559848)
  line L18 (-214.418458, 363.559848) -> (-188.300059, 363.559848)
  arc A3 (-214.418458, 363.559848) -> (-216.243955, 357.78712) centre (-214.418458, 360.384848) ccw
  arc A4 (-357.78712, 216.243955) -> (-216.243955, 357.78712) centre (-274.659848, 274.659848) ccw
  arc A5 (-357.78712, 216.243955) -> (-363.559848, 214.418458) centre (-360.384848, 214.418458) ccw
  line L19 (-363.559848, 188.299848) -> (-363.559848, 214.418458)
  line L20 (-357.209848, 30.819848) -> (-363.559848, 30.819848)
  line L21 (-363.559848, 4.701237) -> (-363.559848, 30.819848)
  arc A6 (-363.559848, 4.701237) -> (-357.78712, 2.87574) centre (-360.384848, 4.701237) ccw
  arc A7 (-216.243955, -138.667425) -> (-357.78712, 2.87574) centre (-274.659848, -55.540152) ccw
  arc A8 (-216.243955, -138.667425) -> (-214.418458, -144.440152) centre (-214.418458, -141.265152) ccw
  line L22 (-188.300059, -144.440152) -> (-214.418458, -144.440152)
  line L23 (-30.820059, -138.090152) -> (-30.820059, -144.440152)
  line L24 (-4.701237, -144.440152) -> (-30.820059, -144.440152)
  arc A9 (-4.701237, -144.440152) -> (-2.87574, -138.667425) centre (-4.701237, -141.265152) ccw
  arc A10 (138.667425, 2.87574) -> (-2.87574, -138.667425) centre (55.540152, -55.540152) ccw
  arc A11 (138.667425, 2.87574) -> (144.440152, 4.701237) centre (141.265152, 4.701237) ccw
  line L25 (144.440152, 30.819848) -> (144.440152, 4.701237)
  line L26 (-188.300059, -144.440152) -> (-30.820059, -144.440152)
  line L27 (-30.820059, -144.440152) -> (-30.820059, -138.090152)
  line L28 (-30.820059, -138.090152) -> (-188.300059, -138.090152)
  line L29 (-188.300059, -138.090152) -> (-188.300059, -144.440152)
  line L30 (144.440152, 30.819848) -> (138.090152, 30.819848)
  line L31 (138.090152, 30.819848) -> (138.090152, 188.299848)
  line L32 (138.090152, 188.299848) -> (144.440152, 188.299848)
  line L33 (144.440152, 188.299848) -> (144.440152, 30.819848)
  line L34 (-188.300059, 363.559848) -> (-30.820059, 363.559848)
  line L35 (-30.820059, 363.559848) -> (-30.820059, 357.209848)
  line L36 (-30.820059, 357.209848) -> (-188.300059, 357.209848)
  line L37 (-188.300059, 357.209848) -> (-188.300059, 363.559848)
  line L38 (-363.559848, 188.299848) -> (-357.209848, 188.299848)
  line L39 (-357.209848, 188.299848) -> (-357.209848, 30.819848)
  line L40 (-357.209848, 30.819848) -> (-363.559848, 30.819848)
  line L41 (-363.559848, 30.819848) -> (-363.559848, 188.299848)
  point P0 (0, 0)
  constraints: 32 end point, 8 parallel, 4 horizontal, 4 perpendicular
extrude "Extrusion14" add sketch "Sketch15" against normal blind 6.35
sketch "Sketch16" plane through (0, 6.35, 0) normal (0, 1, 0) x (1, 0, 0)
  line L0 (-4.701237, -144.440152) -> (-214.418458, -144.440152)
  line L1 (-109.559848, -144.440152) -> (-37.169848, -144.440152)
  line L2 (-37.169848, -144.440152) -> (-181.949848, -144.440152)
  line L3 (-181.949848, -144.440152) -> (-200.999848, -144.440152)
  line L4 (-200.999848, -144.440152) -> (-181.949848, -144.440152)
  line L5 (-181.949848, -144.440152) -> (-181.949848, -131.740152)
  line L6 (-181.949848, -131.740152) -> (-200.999848, -131.740152)
  line L7 (-200.999848, -131.740152) -> (-200.999848, -144.440152)
  line L8 (-37.169848, -144.440152) -> (-18.119848, -144.440152)
  line L9 (-18.119848, -144.440152) -> (-18.119848, -131.740152)
  line L10 (-18.119848, -131.740152) -> (-37.169848, -131.740152)
  line L11 (-37.169848, -131.740152) -> (-37.169848, -144.440152)
  point P0 (0, 0)
  dimension "d116" = 72.39
  dimension "d117" = 144.78
  dimension "d118" = 19.05
  dimension "d119" = 12.7
  dimension "d120" = 19.05
  constraints: 22 end point, 4 parallel, 3 point on line, 2 horizontal, 2 perpendicular, 1 midpoint
  measures "d116" distance of L1.start L1.end
  measures "d117" distance of L1.end L2.end
  measures "d118" distance of L2.end L3.end
  measures "d119" distance of L5.end L4.end
  measures "d120" distance of L10.end L9.end
extrude "Extrusion15" cut sketch "Sketch16" against normal blind 6.35
sketch "Sketch17" plane through (0, 6.35, 0) normal (0, 1, 0) x (1, 0, 0)
  line L0 (-200.999848, -131.740152) -> (-18.119848, -131.740152)
  line L1 (-18.119848, -131.740152) -> (-18.119848, -144.440152)
  line L2 (-18.119848, -144.440152) -> (-200.999848, -144.440152)
  line L3 (-200.999848, -144.440152) -> (-200.999848, -131.740152)
  point P0 (0, 0)
  constraints: 8 end point, 2 parallel, 1 horizontal, 1 perpendicular
extrude "Extrusion16" add sketch "Sketch17" against normal blind 6.35
sketch "Sketch18" plane through (0, 6.35, 0) normal (0, 1, 0) x (1, 0, 0)
  line L0 (-4.701237, -144.440152) -> (-214.418458, -144.440152)
  arc A0 (-4.701237, -144.440152) -> (-2.87574, -138.667425) centre (-4.701237, -141.265152) ccw
  arc A1 (138.667425, 2.87574) -> (-2.87574, -138.667425) centre (55.540152, -55.540152) ccw
  line L1 (-11.661931, -131.740152) -> (-11.661931, -144.440152)
  point P0 (0, 0)
  dimension "d125" = 12.7
  constraints: 2 end point, 1 perpendicular, 1 point on circle, 1 point on line
  measures "d125" distance of L1.start L1.end
extrude "Extrusion17" cut sketch "Sketch18" against normal blind 6.35
sketch "Sketch19" plane through (0, 6.35, 0) normal (0, 1, 0) x (1, 0, 0)
  arc A0 (-216.243955, -138.667425) -> (-357.78712, 2.87574) centre (-274.659848, -55.540152) ccw
  arc A1 (-216.243955, -138.667425) -> (-214.418458, -144.440152) centre (-214.418458, -141.265152) ccw
  line L0 (-11.661931, -144.440152) -> (-214.418458, -144.440152)
  line L1 (-207.457764, -144.440152) -> (-207.457764, -131.740152)
  point P0 (0, 0)
  dimension "d128" = 12.7
  constraints: 2 end point, 1 perpendicular, 1 point on circle, 1 point on line
  measures "d128" distance of L1.start L1.end
extrude "Extrusion18" cut sketch "Sketch19" against normal blind 6.35
sketch "Sketch20" plane through (0, 6.35, 0) normal (0, 1, 0) x (1, 0, 0)
  line L0 (-207.457764, -131.740152) -> (-207.457764, -144.440152)
  line L1 (-11.661931, -144.440152) -> (-207.457764, -144.440152)
  line L2 (-11.661931, -144.440152) -> (-11.661931, -131.740152)
  arc A0 (138.667425, 2.87574) -> (-11.661931, -131.740152) centre (55.540152, -55.540152) ccw
  arc A1 (-207.457764, -131.740152) -> (-357.78712, 2.87574) centre (-274.659848, -55.540152) ccw
  line L3 (-109.559848, -144.440152) -> (-11.769848, -144.440152)
  line L4 (-11.769848, -144.440152) -> (-207.349848, -144.440152)
  line L5 (-207.349848, -144.440152) -> (-207.349848, -131.644843)
  line L6 (-11.769848, -144.440152) -> (-11.769848, -131.644843)
  point P0 (0, 0)
  dimension "d131" = 97.79
  dimension "d132" = 195.58
  constraints: 8 end point, 2 point on circle, 2 point on line, 1 midpoint, 1 parallel, 1 perpendicular
  measures "d131" distance of L3.start L3.end
  measures "d132" distance of L3.end L4.end
extrude "Extrusion19" cut sketch "Sketch20" against normal blind 6.35
sketch "Sketch21" plane through (0, 6.35, 0) normal (0, 1, 0) x (1, 0, 0)
  arc A0 (138.667425, 2.87574) -> (-11.769848, -131.644843) centre (55.540152, -55.540152) ccw
  arc A1 (138.667425, 2.87574) -> (144.440152, 4.701237) centre (141.265152, 4.701237) ccw
  line L0 (144.440152, 214.418458) -> (144.440152, 4.701237)
  arc A2 (144.440152, 214.418458) -> (138.667425, 216.243955) centre (141.265152, 214.418458) ccw
  arc A3 (-2.87574, 357.78712) -> (138.667425, 216.243955) centre (55.540152, 274.659848) ccw
  arc A4 (-2.87574, 357.78712) -> (-4.701237, 363.559848) centre (-4.701237, 360.384848) ccw
  line L1 (-214.418458, 363.559848) -> (-4.701237, 363.559848)
  arc A5 (-214.418458, 363.559848) -> (-216.243955, 357.78712) centre (-214.418458, 360.384848) ccw
  arc A6 (-357.78712, 216.243955) -> (-216.243955, 357.78712) centre (-274.659848, 274.659848) ccw
  arc A7 (-357.78712, 216.243955) -> (-363.559848, 214.418458) centre (-360.384848, 214.418458) ccw
  line L2 (-363.559848, 4.701237) -> (-363.559848, 214.418458)
  arc A8 (-363.559848, 4.701237) -> (-357.78712, 2.87574) centre (-360.384848, 4.701237) ccw
  arc A9 (-207.349848, -131.644843) -> (-357.78712, 2.87574) centre (-274.659848, -55.540152) ccw
  line L3 (-207.349848, 350.764538) -> (-207.349848, 363.559848)
  line L4 (-11.769848, 363.559848) -> (-11.769848, 350.764538)
  line L5 (144.440152, 109.559848) -> (144.440152, 207.349848)
  line L6 (144.440152, 207.349848) -> (131.644843, 207.349848)
  line L7 (144.440152, 207.349848) -> (144.440152, 11.769848)
  line L8 (144.440152, 11.769848) -> (131.644843, 11.769848)
  line L9 (-363.559848, 11.769848) -> (-350.764538, 11.769848)
  line L10 (-363.559848, 207.349848) -> (-350.764538, 207.349848)
  point P0 (0, 0)
  dimension "d135" = 97.79
  dimension "d136" = 195.58
  constraints: 16 end point, 6 point on circle, 6 point on line, 4 perpendicular, 2 equal length, 1 midpoint
  measures "d135" distance of L5.start L5.end
  measures "d136" distance of L5.end L7.end
extrude "Extrusion20" cut sketch "Sketch21" against normal blind 25.4
sketch "Sketch22" plane through (0, 0, 0) normal (0, -1, 0) x (1, 0, 0)
  line L0 (144.440152, 144.440152) -> (-84.159848, 144.440152)
  line L1 (-84.159848, 144.440152) -> (-84.159848, -51.139848)
  line L2 (-84.159848, -51.139848) -> (144.440152, -51.139848)
  line L3 (144.440152, -51.139848) -> (144.440152, 144.440152)
  line L4 (-363.559848, 144.440152) -> (-134.959848, 144.440152)
  line L5 (-134.959848, 144.440152) -> (-134.959848, -51.139848)
  line L6 (-134.959848, -51.139848) -> (-363.559848, -51.139848)
  line L7 (-363.559848, -51.139848) -> (-363.559848, 144.440152)
  line L8 (-134.959848, -51.139848) -> (-147.659848, -51.139848)
  line L9 (-147.659848, -51.139848) -> (-147.659848, -25.739848)
  line L10 (-147.659848, -25.739848) -> (-134.959848, -25.739848)
  line L11 (-134.959848, -25.739848) -> (-134.959848, -51.139848)
  line L12 (-84.159848, -51.139848) -> (-71.459848, -51.139848)
  line L13 (-71.459848, -51.139848) -> (-71.459848, -25.739848)
  line L14 (-71.459848, -25.739848) -> (-84.159848, -25.739848)
  line L15 (-84.159848, -25.739848) -> (-84.159848, -51.139848)
  point P0 (0, 0)
  dimension "d139" = 228.6
  dimension "d140" = 195.58
  dimension "d141" = 228.6
  dimension "d142" = 12.7
  dimension "d143" = 25.4
  dimension "d144" = 12.7
  dimension "d145" = 25.4
  constraints: 32 end point, 8 parallel, 4 horizontal, 4 perpendicular
  measures "d139" distance of L2.end L1.end
  measures "d140" distance of L1.end L0.end
  measures "d141" distance of L5.end L6.end
  measures "d142" distance of L9.end L10.end
  measures "d143" distance of L8.end L9.end
  measures "d144" distance of L14.end L13.end
  measures "d145" distance of L13.end L12.end
extrude "Extrusion21" cut sketch "Sketch22" against normal blind 25.4 contours L14 L13 L2 L1 | L5 L6 L9 L10
body "Solid1"
